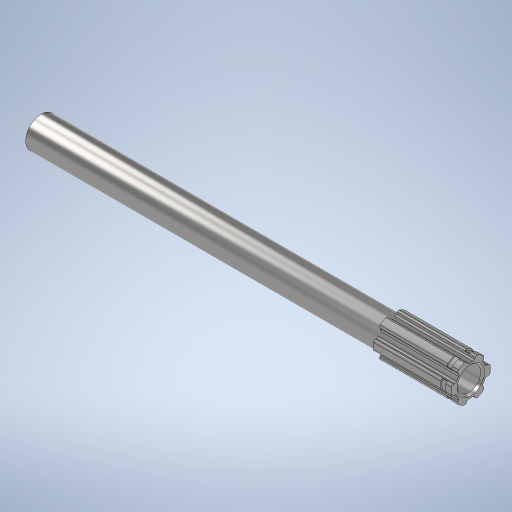
# Autodesk Inventor part: Shaft
Saved by Autodesk Inventor 2023.2 (Build 272271000, 271)
## iProperties
Created: 2024-01-10
Part Number: Shaft
Material: Stainless Steel
Document SubType Name: Modeling
Designer: Nathan Cai
Density: 8 g/cm^3
Appearance: Semi-Polished
Mass: 19.5086 g
Surface Area: 45.8372 cm^2
Volume: 2.43857 cm^3
Author: Nathan Cai
Autodesk Inventor part; units mm, degrees
ref_plane "YZ Plane" through (0, 0, 0) normal (1, 0, 0) x (0, 1, 0)
ref_plane "XZ Plane" through (0, 0, 0) normal (0, 1, 0) x (-1, 0, 0)
sketch "Sketch1" plane through (0, 0, 0) normal (1, 0, 0) x (0, 1, 0)
  circle A0 centre (0, 0) radius 3.95
  circle A1 centre (0, 0) radius 3
  dimension "d0" = 7.9
  dimension "d1" = 6
  constraints: 2 centre point, 2 coincident
  measures "d0" diameter of A0
  measures "d1" diameter of A1
extrude "Extrusion1" add sketch "Sketch1" along normal blind 110
sketch "Sketch2" plane through (110, 0, 0) normal (1, 0, 0) x (0, 0, -1)
  line L0 (-0.0955, 0) -> (3.95, 0) construction
  circle A0 centre (0, 0) radius 3.95 projected
  line L1 (4.8412, 1.25) -> (0, 1.25)
  line L2 (0, 1.25) -> (0, -1.25) construction
  line L3 (0, -1.25) -> (4.8412, -1.25)
  line L4 (4.8412, -1.25) -> (4.8412, 1.25) construction
  line L5 (4.8412, 1.25) -> (0, -1.25) construction
  line L6 (0, 1.25) -> (4.8412, -1.25) construction
  circle A1 centre (0, 0) radius 5
  line L7 (-0.0477, -0.0827) -> (1.975, 3.4208) construction
  line L8 (1.3381, 4.8176) -> (-1.0825, 0.625)
  line L9 (-1.0825, 0.625) -> (1.0825, -0.625) construction
  line L10 (1.0825, -0.625) -> (3.5031, 3.5676)
  line L11 (3.5031, 3.5676) -> (1.3381, 4.8176) construction
  line L12 (1.3381, 4.8176) -> (1.0825, -0.625) construction
  line L13 (-1.0825, 0.625) -> (3.5031, 3.5676) construction
  line L14 (0.0477, -0.0827) -> (-1.975, 3.4208) construction
  line L15 (-3.5031, 3.5676) -> (-1.0825, -0.625)
  line L16 (-1.0825, -0.625) -> (1.0825, 0.625) construction
  line L17 (1.0825, 0.625) -> (-1.3381, 4.8176)
  line L18 (-1.3381, 4.8176) -> (-3.5031, 3.5676) construction
  line L19 (-3.5031, 3.5676) -> (1.0825, 0.625) construction
  line L20 (-1.0825, -0.625) -> (-1.3381, 4.8176) construction
  line L21 (0.0955, 0) -> (-3.95, 0) construction
  line L22 (-4.8412, -1.25) -> (0, -1.25)
  line L23 (0, -1.25) -> (0, 1.25) construction
  line L24 (0, 1.25) -> (-4.8412, 1.25)
  line L25 (-4.8412, 1.25) -> (-4.8412, -1.25) construction
  line L26 (-4.8412, -1.25) -> (0, 1.25) construction
  line L27 (0, -1.25) -> (-4.8412, 1.25) construction
  line L28 (0.0477, 0.0827) -> (-1.975, -3.4208) construction
  line L29 (-1.3381, -4.8176) -> (1.0825, -0.625)
  line L30 (1.0825, -0.625) -> (-1.0825, 0.625) construction
  line L31 (-1.0825, 0.625) -> (-3.5031, -3.5676)
  line L32 (-3.5031, -3.5676) -> (-1.3381, -4.8176) construction
  line L33 (-1.3381, -4.8176) -> (-1.0825, 0.625) construction
  line L34 (1.0825, -0.625) -> (-3.5031, -3.5676) construction
  line L35 (-0.0477, 0.0827) -> (1.975, -3.4208) construction
  line L36 (3.5031, -3.5676) -> (1.0825, 0.625)
  line L37 (1.0825, 0.625) -> (-1.0825, -0.625) construction
  line L38 (-1.0825, -0.625) -> (1.3381, -4.8176)
  line L39 (1.3381, -4.8176) -> (3.5031, -3.5676) construction
  line L40 (3.5031, -3.5676) -> (-1.0825, -0.625) construction
  line L41 (1.0825, 0.625) -> (1.3381, -4.8176) construction
  point P0 (2.4206, 0)
  point P1 (1.2103, 2.0963)
  point P2 (-1.2103, 2.0963)
  point P3 (-2.4206, 0)
  point P4 (-1.2103, -2.0963)
  point P5 (1.2103, -2.0963)
  point P6 (-2.956, -2.62)
  point P7 (-3.5031, -3.5676)
  point P8 (-1.3381, -4.8176)
  point P9 (-0.791, -3.87)
  point P10 (0.791, -3.87)
  point P11 (1.3381, -4.8176)
  point P12 (3.5031, -3.5676)
  point P13 (2.956, -2.62)
  point P14 (4.8412, 1.25)
  point P15 (3.747, 1.25)
  point P16 (3.747, -1.25)
  point P17 (2.956, 2.62)
  point P18 (3.5031, 3.5676)
  point P19 (1.3381, 4.8176)
  point P20 (0.791, 3.87)
  point P21 (-3.747, 1.25)
  point P22 (-4.8412, -1.25)
  point P23 (-3.747, -1.25)
  point P24 (-0.791, 3.87)
  point P25 (-1.3381, 4.8176)
  point P26 (-3.5031, 3.5676)
  point P27 (-2.956, 2.62)
  dimension "d23" = 10
  dimension "d21" = 2.5
  dimension "d26" = 360
  constraints: 84 end point, 18 midpoint, 12 point on line, 8 coincident, 3 parallel, 1 horizontal, 1 perpendicular, 106 other
  measures "d21" distance of L2.end L1.end
extrude "Extrusion2" add sketch "Sketch2" against normal blind 20 contours A0 L1 A1 L3 | A0 L8 A1 L10 | L36 A1 L38 A0 | A0 L15 A1 L17 | L29 A1 L31 A0 | A0 L22 A1 L24
fillet "Fillet1" radius 0.5 24 edges at (100, 4.8176, 1.3381) (100, 3.5676, 3.5031) (100, 4.8176, -1.3381) (100, 3.5676, -3.5031) (100, 1.25, -4.8412) (100, -1.25, -4.8412) (100, -3.5676, -3.5031) (100, -4.8176, -1.3381) (100, -4.8176, 1.3381) (100, -3.5676, 3.5031) (100, -1.25, 4.8412) (100, 1.25, 4.8412) (100, 3.87, -0.791) (100, 3.87, 0.791) (100, 2.62, -2.956) (100, 1.25, -3.747) (100, -1.25, -3.747) (100, -2.62, -2.956) (100, -3.87, -0.791) (100, -3.87, 0.791) (100, -2.62, 2.956) (100, -1.25, 3.747) (100, 1.25, 3.747) (100, 2.62, 2.956)
ref_plane "Work Plane1" through (108.5, 0, 0) normal (1, 0, 0) x (0, 0, -1)
sketch "Sketch4" plane through (108.5, 0, 0) normal (1, 0, 0) x (0, 0, -1)
  arc A0 (3.6317, -1.5534) -> (3.6317, 1.5534) centre (0, 0) ccw projected
  circle A1 centre (0, 0) radius 10
  circle A2 centre (0, 0) radius 4.7
  arc A3 (0.4706, 3.9219) -> (-0.4706, 3.9219) centre (0, 0) ccw projected
  point P0 (5.7956, 1.5529)
  point P1 (5.7956, -1.5529)
  point P2 (6, 0)
  point P3 (3.747, -1.25)
  point P4 (3.747, 1.25)
  dimension "d14" = 20
  dimension "d29" = 9.4
  constraints: 2 centre point, 2 coincident, 3 other
  measures "d14" diameter of A1
  measures "d29" diameter of A2
extrude "Extrusion4" cut sketch "Sketch4" against normal blind 1.2
chamfer "Chamfer1" distance 0.5 angle 45 1 edges at (110, -3, 0)
sketch "Sketch3" plane through (0, 0, 0) normal (0, 1, 0) x (-1, 0, 0)
  line L0 (0, 0) -> (-110, 0) construction
  line L1 (-110, -3) -> (-110, 3) projected
  circle A0 centre (-3.95, 0) radius 1.5
  circle A1 centre (-3.95, 0) radius 3.95
  line L2 (0, 3.95) -> (-90, 3.95) projected
  line L3 (0, 3.95) -> (0, -3.95) projected
  line L4 (-7.9, -3.95) -> (0, -3.95)
  line L5 (0, -3.95) -> (0, 3.95)
  line L6 (0, 3.95) -> (-7.9, 3.95)
  line L7 (-7.9, 3.95) -> (-7.9, -3.95)
  line L8 (-7.9, -3.95) -> (0, 3.95) construction
  line L9 (0, -3.95) -> (-7.9, 3.95) construction
  point P0 (-3.95, 3.95)
  point P1 (-3.95, -3.95)
  point P2 (0, -3.95)
  dimension "d10" = 3
  constraints: 14 end point, 3 midpoint, 2 centre point, 2 parallel, 2 tangent, 1 coincident, 1 horizontal, 1 perpendicular, 1 point on line
  measures "d10" diameter of A0
sketch "Sketch5" plane through (0, 0, 0) normal (0, 0, 1) x (1, 0, 0)
  line L0 (0, -3.95) -> (0, 3.95) projected
  line L1 (90, 2.3685) -> (110, 2.3685) projected
  line L2 (90, 2.3685) -> (90, 3.9219) projected
  line L3 (110, 3.9219) -> (90, 3.9219) projected
  line L4 (110, 3.9219) -> (110, 3.9219) projected
  line L5 (90, 3.9219) -> (110, 3.9219) projected
  line L6 (90, 3.9219) -> (90, 2.3685) projected
  line L7 (110, 2.3685) -> (90, 2.3685) projected
  line L8 (110, 1.5534) -> (110, 2.3685) projected
  line L9 (90, 1.5534) -> (110, 1.5534) projected
  line L10 (90, 1.5534) -> (90, -1.5534) projected
  line L11 (110, -1.5534) -> (90, -1.5534) projected
  line L12 (110, -2.3685) -> (110, -1.5534) projected
  line L13 (90, -2.3685) -> (110, -2.3685) projected
  line L14 (90, -2.3685) -> (90, -3.9219) projected
  line L15 (110, -3.9219) -> (90, -3.9219) projected
  line L16 (110, -3.9219) -> (110, -3.9219) projected
  line L17 (90, -3.9219) -> (110, -3.9219) projected
  line L18 (90, -3.9219) -> (90, -2.3685) projected
  line L19 (110, -2.3685) -> (90, -2.3685) projected
  line L20 (110, -1.5534) -> (110, -2.3685) projected
  line L21 (90, -1.5534) -> (110, -1.5534) projected
  line L22 (90, -1.5534) -> (90, 1.5534) projected
  line L23 (110, 1.5534) -> (90, 1.5534) projected
  line L24 (110, 2.3685) -> (110, 1.5534) projected
  line L25 (3.95, 3.6541) -> (3.95, -3.6541) construction
  line L26 (3.95, -3.6541) -> (3.95, 3.6541)
  line L27 (2.45, 0) -> (5.45, 0) construction
  line L28 (2.45, -2) -> (5.45, -2)
  line L29 (5.45, 2) -> (2.45, 2)
  arc A0 (2.45, 2) -> (2.45, -2) centre (2.45, 0) ccw
  arc A1 (5.45, -2) -> (5.45, 2) centre (5.45, 0) ccw
  line L30 (-2.45, 2) -> (2.45, 2)
  line L31 (2.45, 2) -> (2.45, -2)
  line L32 (2.45, -2) -> (-2.45, -2)
  line L33 (-2.45, -2) -> (-2.45, 2)
  line L34 (-2.45, 2) -> (2.45, -2) construction
  line L35 (2.45, 2) -> (-2.45, -2) construction
  point P0 (0, 0)
  point P1 (3.95, 0)
  dimension "d30" = 4
  dimension "d31" = 3
  constraints: 24 end point, 4 equal length, 4 midpoint, 4 point on circle, 4 tangent, 2 centre point, 2 perpendicular, 1 horizontal, 1 vertical
  measures "d30" diameter of A1
  measures "d31" distance of L27.start L27.end
body "Solid1"
